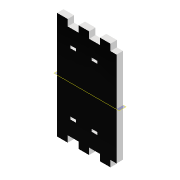
# Autodesk Inventor part: 00_Baseplate_Simmo_side6_v2
Saved by Autodesk Inventor 2022.5 (Build 265521000, 521)
## iProperties
Created: 2022-08-09
Part Number: 00_Baseplate_Simmo_side6_v2
Material: Generic
Document SubType Name: Modeling
Designer: wanghaoran
Density: 1 g/cm^3
Appearance: Default
Author: wanghaoran
Autodesk Inventor part; units mm, degrees
ref_plane "YZ Plane" through (0, 0, 0) normal (1, 0, 0) x (0, 1, 0)
ref_plane "XZ Plane" through (0, 0, 0) normal (0, 1, 0) x (-1, 0, 0)
ref_plane "XY Plane" through (0, 0, 0) normal (0, 0, 1) x (1, 0, 0)
sketch "Sketch1" plane through (0, 0, 0) normal (0, 0, 1) x (1, 0, 0)
  line L0 (50, 11) -> (55.5309, 11) projected
  line L1 (0, 11) -> (0, 17) projected
  line L2 (0, 11) -> (0, 17) projected
  line L3 (0, 11) -> (0, 17) projected
  line L4 (0, 17) -> (55.5309, 17)
  line L5 (55.5309, 17) -> (55.5309, -83)
  line L6 (55.5309, -83) -> (0, -83)
  line L7 (0, -83) -> (0, 17)
  line L8 (55.5309, 17) -> (55.5309, 11) projected
  line L9 (55.5309, 17) -> (55.5309, 11) projected
  dimension "d16" = 100
  constraints: 8 end point, 2 parallel, 1 horizontal, 1 perpendicular
  measures "d16" distance of L4.end L5.end
extrude "Extrusion1" add sketch "Sketch1" along normal blind 6
sketch "Sketch2" plane through (0, 0, 6) normal (0, 0, 1) x (1, 0, 0)
  line L0 (50, 11) -> (55.5309, 11) projected
  line L1 (50, 17) -> (50, 11) projected
  line L2 (30, 17) -> (30, 11) projected
  line L3 (30, 11) -> (40, 11) projected
  line L4 (40, 11) -> (40, 17) projected
  line L5 (50, 11) -> (49.9, 11)
  line L6 (49.9, 11) -> (49.9, 17)
  line L7 (49.9, 17) -> (50, 17)
  line L8 (50, 17) -> (50, 11)
  line L9 (40, 11) -> (40.1, 11)
  line L10 (40.1, 11) -> (40.1, 17)
  line L11 (40.1, 17) -> (40, 17)
  line L12 (40, 17) -> (40, 11)
  line L13 (30, 11) -> (29.9, 11)
  line L14 (29.9, 11) -> (29.9, 17)
  line L15 (29.9, 17) -> (30, 17)
  line L16 (30, 17) -> (30, 11)
  line L17 (10, 17) -> (10, 11) projected
  line L18 (20, 11) -> (20, 17) projected
  line L19 (10, 11) -> (20, 11) projected
  line L20 (20, 11) -> (20.1, 11)
  line L21 (20.1, 11) -> (20.1, 17)
  line L22 (20.1, 17) -> (20, 17)
  line L23 (20, 17) -> (20, 11)
  line L24 (10, 11) -> (9.9, 11)
  line L25 (9.9, 11) -> (9.9, 17)
  line L26 (9.9, 17) -> (10, 17)
  line L27 (10, 17) -> (10, 11)
  line L28 (55.5309, -83) -> (55.5309, 17) projected
  line L29 (40, 11) -> (30, 11)
  line L30 (20, 11) -> (10, 11)
  line L31 (50, 11) -> (55.5309, 11)
  line L32 (0, 17) -> (0, -83) projected
  line L33 (55.5309, 17) -> (0, 17)
  point P0 (49.9, 0.06)
  point P1 (30.1, 0)
  point P2 (39.9, 0)
  point P3 (39.9, 0.03)
  point P4 (30.1, 2.97)
  point P5 (40, 0)
  point P6 (40, 0)
  dimension "d3" = 0.1
  dimension "d4" = 6
  dimension "d5" = 0.1
  dimension "d6" = 6
  dimension "d7" = 0.1
  dimension "d8" = 6
  dimension "d17" = 0.1
  dimension "d18" = 6
  dimension "d19" = 0.1
  dimension "d20" = 6
  constraints: 48 end point, 13 equal length, 6 horizontal, 5 perpendicular
  measures "d3" distance of L6.end L7.end
  measures "d4" distance of L5.end L6.end
  measures "d5" distance of L11.end L10.end
  measures "d6" distance of L10.end L9.end
  measures "d7" distance of L14.end L15.end
  measures "d8" distance of L13.end L14.end
  measures "d17" distance of L22.end L21.end
  measures "d18" distance of L21.end L20.end
  measures "d19" distance of L25.end L26.end
  measures "d20" distance of L24.end L25.end
extrude "Extrusion2" cut sketch "Sketch2" against normal through all contours L1 L33 L28 L0 | L5 L6 L7 L1 | L33 L4 L3 L2 | L2 L13 L14 L15 | L33 L18 L19 L17 | L17 L24 L25 L26 | L22 L21 L20 L18
ref_plane "Work Plane1" through (0, -33, 0) normal (0, -1, 0) x (1, 0, 0)
mirror "Mirror1" about plane through (0, -33, 0) normal (0, -1, 0) of "Extrusion2"
sketch "Sketch3" plane through (0, 0, 6) normal (0, 0, 1) x (1, 0, 0)
  line L0 (37.75, -5.4) -> (32.25, -5.4)
  line L1 (32.25, -5.4) -> (32.25, -3)
  line L2 (32.25, -3) -> (37.75, -3)
  line L3 (37.75, -3) -> (37.75, -5.4)
  line L4 (40.1, 7.6673) -> (40.1, 6) projected
  line L5 (40.1, 0) -> (29.9, 0) projected
  point P0 (0, 0)
  dimension "d21" = 5.5
  dimension "d22" = 2.4
  dimension "d23" = 2.35
  dimension "d24" = 3
  constraints: 8 end point, 2 parallel, 1 horizontal, 1 perpendicular
  measures "d21" distance of L1.end L2.end
  measures "d22" distance of L0.end L1.end
  measures "d23" distance between parallel lines of L4 L3
  measures "d24" distance between parallel lines of L5 L2
extrude "Extrusion3" cut sketch "Sketch3" against normal through all
pattern_linear "Rectangular Pattern1" count 2 spacing 20 along (-1, 0, 0) of "Extrusion3"
mirror "Mirror2" about plane through (0, -33, 0) normal (0, -1, 0) of "Extrusion3", "Rectangular Pattern1"
body "Solid1"
